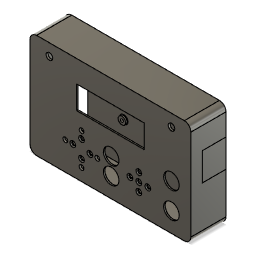
MegaElsCase (Autodesk Fusion 360 design; units mm, degrees)
Autodesk Fusion 360 part; units mm, degrees
sketch "Sketch1" plane through (0, 0, 0) normal (0, 0, 1) x (1, 0, 0)
  line L0 (0, 0) -> (160, 0)
  line L1 (160, 0) -> (160, 100)
  line L2 (160, 100) -> (0, 100)
  line L3 (0, 100) -> (0, 0)
  dimension "d1" = 160
  dimension "d2" = 100
  constraint horizontal L0
  constraint vertical L1
  constraint horizontal L2
  constraint vertical L3
  constraint coincident L0.start L3.end
  measures "d1" distance of L0.start L0.end
  measures "d2" distance of L0.start L2.end
extrude "Extrude1" add sketch "Sketch1" along normal blind 1.6 makes body 1
sketch "Sketch2" plane through (0, 0, 1.6) normal (0, 0, 1) x (1, 0, 0)
  line L0 (0, 100) -> (0, 0)
  line L1 (0, 0) -> (160, 0)
  line L2 (160, 0) -> (160, 100)
  line L3 (160, 100) -> (0, 100)
  line L4 (0, 0) -> (160, 0)
  line L5 (160, 0) -> (160, 100)
  line L6 (160, 100) -> (0, 100)
  line L7 (0, 100) -> (0, 0)
  line L8 (163, 103) -> (-3, 103)
  line L9 (-3, 103) -> (-3, -3)
  line L10 (-3, -3) -> (163, -3)
  line L11 (163, -3) -> (163, 103)
  line L12 (165, 105) -> (-5, 105)
  line L13 (-5, 105) -> (-5, -5)
  line L14 (-5, -5) -> (165, -5)
  line L15 (165, -5) -> (165, 105)
  circle A0 centre (15.5185, 92.5006) radius 3.5
  circle A1 centre (144.5011, 92.3883) radius 3.5
  circle A2 centre (80.8196, 33.8708) radius 8.25
  circle A3 centre (80.8007, 15.6853) radius 8.25
  circle A4 centre (144.4573, 43.0009) radius 8.25
  circle A5 centre (144.4275, 15.6835) radius 8.25
  line L16 (44.3, 81.7) -> (115.7, 81.7)
  line L17 (115.7, 81.7) -> (115.7, 57.3)
  line L18 (115.7, 57.3) -> (44.3, 57.3)
  line L19 (44.3, 57.3) -> (44.3, 81.7)
  circle A6 centre (49.4839, 33.8731) radius 2
  circle A7 centre (40.2387, 24.6612) radius 2
  circle A8 centre (58.3342, 24.6842) radius 2
  circle A9 centre (49.4706, 15.6511) radius 2
  circle A10 centre (49.4462, 7.8513) radius 2.5
  circle A11 centre (66.167, 24.6779) radius 2.5
  circle A12 centre (49.495, 41.543) radius 2.5
  circle A13 centre (32.3413, 24.6561) radius 2.5
  circle A14 centre (109.969, 33.8254) radius 2
  circle A15 centre (100.5787, 24.7006) radius 2
  circle A16 centre (109.9576, 24.7062) radius 2
  circle A17 centre (119.4752, 24.7124) radius 2
  circle A18 centre (109.9462, 15.6346) radius 2
  line L20 (32.3413, 24.6561) -> (119.4752, 24.7124) construction
  line L21 (49.495, 41.543) -> (49.4462, 7.8513) construction
  line L22 (109.969, 33.8254) -> (109.9462, 15.6346) construction
  circle A19 centre (2.54, 97.46) radius 2
  circle A20 centre (157.46, 97.46) radius 2
  circle A21 centre (157.46, 2.54) radius 2
  circle A22 centre (2.54, 2.54) radius 2
  circle A23 centre (2.54, 97.46) radius 4
  circle A24 centre (2.54, 2.54) radius 4
  circle A25 centre (157.46, 2.54) radius 4
  circle A26 centre (157.46, 97.46) radius 4
  line L23 (157.46, 6.54) -> (163, 6.54)
  line L24 (153.46, 2.54) -> (153.46, -3)
  line L25 (6.54, 2.54) -> (6.54, -3)
  line L26 (2.54, 6.54) -> (-3, 6.54)
  line L27 (2.54, 93.46) -> (-3, 93.46)
  line L28 (6.54, 97.46) -> (6.54, 103)
  line L29 (153.46, 97.46) -> (153.46, 103)
  line L30 (157.46, 93.46) -> (163, 93.46)
  circle A27 centre (100, 40) radius 2
  circle A28 centre (60, 40) radius 2
  circle A29 centre (60, 40) radius 4
  circle A30 centre (100, 40) radius 4
  line L31 (155.46, 100.9241) -> (155.46, 103)
  line L32 (160.9241, 95.46) -> (163, 95.46)
  line L33 (4.54, 100.9241) -> (4.54, 103)
  line L34 (-0.9241, 95.46) -> (-3, 95.46)
  line L35 (-0.9241, 4.54) -> (-3, 4.54)
  line L36 (4.54, -0.9241) -> (4.54, -3)
  line L37 (155.46, -0.9241) -> (155.46, -3)
  line L38 (160.9241, 4.54) -> (163, 4.54)
  dimension "d5" = 3
  dimension "d6" = 5
  dimension "d7" = 7
  dimension "d8" = 7
  dimension "d9" = 16.5
  dimension "d10" = 16.5
  dimension "d11" = 16.5
  dimension "d12" = 16.5
  dimension "d13" = 18.3
  dimension "d14" = 44.3
  dimension "d15" = 44.3
  dimension "d16" = 24.4
  dimension "d17" = 4
  dimension "d18" = 4
  dimension "d19" = 4
  dimension "d20" = 4
  dimension "d21" = 5
  dimension "d22" = 5
  dimension "d23" = 5
  dimension "d24" = 5
  dimension "d25" = 4
  dimension "d26" = 4
  dimension "d27" = 4
  dimension "d28" = 4
  dimension "d29" = 4
  dimension "d36" = 4
  dimension "d37" = 2.54
  dimension "d38" = 2.54
  dimension "d39" = 4
  dimension "d40" = 2.54
  dimension "d41" = 2.54
  dimension "d42" = 4
  dimension "d43" = 2.54
  dimension "d44" = 2.54
  dimension "d45" = 4
  dimension "d46" = 2.54
  dimension "d47" = 2.54
  dimension "d48" = 2
  dimension "d49" = 2
  dimension "d50" = 2
  dimension "d51" = 2
  dimension "d59" = 4
  dimension "d60" = 4
  dimension "d61" = 2
  dimension "d62" = 2
  dimension "d63" = 60
  dimension "d64" = 60
  dimension "d65" = 60
  dimension "d66" = 100
  dimension "d141" = 2
  dimension "d142" = 2
  dimension "d143" = 2
  dimension "d144" = 2
  dimension "d145" = 2
  dimension "d146" = 2
  dimension "d147" = 2
  dimension "d148" = 2
  constraint horizontal L4
  constraint vertical L5
  constraint horizontal L6
  constraint vertical L7
  constraint coincident L2.end L3.start
  constraint coincident L0.end L1.start
  constraint horizontal L16
  constraint vertical L17
  constraint horizontal L18
  constraint vertical L19
  constraint coincident A13.centre L20.start
  constraint coincident A17.centre L20.end
  constraint coincident A7.centre L20
  constraint coincident A11.centre L20
  constraint coincident A16.centre L20
  constraint coincident A12.centre L21.start
  constraint coincident A10.centre L21.end
  constraint coincident A6.centre L21
  constraint coincident A14.centre L22.start
  constraint coincident A18.centre L22.end
  constraint coincident A16.centre L22
  constraint coincident A25 L23.start
  constraint coincident L11 L23.end
  constraint tangent A25 L23
  constraint horizontal L23
  constraint coincident A25 L24.start
  constraint coincident L10 L24.end
  constraint perpendicular L10 L24
  constraint tangent A25 L24
  constraint coincident A24 L25.start
  constraint coincident L10 L25.end
  constraint coincident A24 L26.start
  constraint coincident L9 L26.end
  constraint perpendicular L9 L26
  constraint tangent A24 L26
  constraint tangent A24 L25
  constraint vertical L25
  constraint coincident A23 L27.start
  constraint coincident L9 L27.end
  constraint perpendicular L9 L27
  constraint coincident A23 L28.start
  constraint coincident L8 L28.end
  constraint perpendicular L8 L28
  constraint tangent A23 L28
  constraint tangent A23 L27
  constraint coincident A26 L29.start
  constraint coincident L8 L29.end
  constraint perpendicular L8 L29
  constraint coincident A26 L30.start
  constraint coincident L11 L30.end
  constraint perpendicular L11 L30
  constraint tangent A26 L30
  constraint tangent A26 L29
  constraint coincident A26 L31.start
  constraint coincident L8 L31.end
  constraint perpendicular L8 L31
  constraint coincident A26 L32.start
  constraint coincident L11 L32.end
  constraint perpendicular L11 L32
  constraint coincident A23 L33.start
  constraint coincident L8 L33.end
  constraint perpendicular L8 L33
  constraint coincident A23 L34.start
  constraint coincident L9 L34.end
  constraint perpendicular L9 L34
  constraint coincident A24 L35.start
  constraint coincident L9 L35.end
  constraint perpendicular L9 L35
  constraint coincident A24 L36.start
  constraint coincident L10 L36.end
  constraint perpendicular L10 L36
  constraint coincident A25 L37.start
  constraint coincident L10 L37.end
  constraint perpendicular L10 L37
  constraint coincident A25 L38.start
  constraint coincident L11 L38.end
  constraint perpendicular L11 L38
  measures "d7" diameter of A0
  measures "d8" diameter of A1
  measures "d9" diameter of A2
  measures "d10" diameter of A3
  measures "d11" diameter of A4
  measures "d12" diameter of A5
  measures "d13" distance of L6 L16
  measures "d14" distance of L7 L19
  measures "d15" distance of L5 L17
  measures "d16" distance of L16 L18
  measures "d17" diameter of A6
  measures "d18" diameter of A7
  measures "d19" diameter of A8
  measures "d20" diameter of A9
  measures "d21" diameter of A10
  measures "d22" diameter of A11
  measures "d23" diameter of A12
  measures "d24" diameter of A13
  measures "d25" diameter of A14
  measures "d26" diameter of A15
  measures "d27" diameter of A16
  measures "d28" diameter of A17
  measures "d29" diameter of A18
  measures "d36" diameter of A19
  measures "d37" distance of L6 A19.centre
  measures "d38" distance of L7 A19.centre
  measures "d39" diameter of A20
  measures "d40" distance of L6 A20.centre
  measures "d41" distance of L5 A20.centre
  measures "d42" diameter of A21
  measures "d43" distance of L5 A21.centre
  measures "d44" distance of L4 A21.centre
  measures "d45" diameter of A22
  measures "d46" distance of L4 A22.centre
  measures "d47" distance of L7 A22.centre
  measures "d48" distance of A19
  measures "d49" distance of A22
  measures "d50" distance of A21
  measures "d51" distance of A20
  measures "d59" diameter of A27
  measures "d60" diameter of A28
  measures "d61" distance of A28
  measures "d62" distance of A27
  measures "d63" distance of L5 A27.centre
  measures "d64" distance of L6 A27.centre
  measures "d65" distance of L6 A28.centre
  measures "d66" distance of L5 A28.centre
  measures "d141" distance of L30 L32
  measures "d142" distance of L29 L31
  measures "d143" distance of L27 L34
  measures "d144" distance of L28 L33
  measures "d145" distance of L26 L35
  measures "d146" distance of L25 L36
  measures "d147" distance of L23 L38
  measures "d148" distance of L24 L37
extrude "Extrude2" add sketch "Sketch2" along normal blind 2 from surface at 8.5 separate body contours L0 L3 L6 L7 A23 | L0 L3 L6 L7 A23 | L0 L7 A23 L27 | L0 L7 L9 A23 L27 L34 | L3 L6 L8 A23 L28 L33 | L3 L6 A23 L28 | L0 L1 L2 L3 L4 L5 L6 L7 A23 A24 A25 A26 L23 L24 L25 L26 L27 L28 L29 L30 | L0 L7 L9 L26 L27 | L8 L9 A23 L33 L34 | L3 L6 L8 L28 L29 | L0 L7 A24 L26 | L0 L7 L9 A24 L26 L35 | L3 L6 L8 A26 L29 L31 | L3 L6 A26 L29 | L0 L1 L4 L7 A24 | L0 L1 L4 L7 A24 | L2 L3 L5 L6 A26 | L2 L3 L5 L6 A26 | L9 L10 A24 L35 L36 | L1 L4 A24 L25 | L8 L11 A26 L31 L32 | L2 L5 A26 L30 | L1 L4 L10 A24 L25 L36 | L1 L4 L10 L24 L25 | L2 L5 L11 A26 L30 L32 | L2 L5 L11 L23 L30 | L1 L4 A25 L24 | L1 L4 L10 A25 L24 L37 | L2 L5 L11 A25 L23 L38 | L2 L5 A25 L23 | L1 L2 L4 L5 A25 | L1 L2 L4 L5 A25 | L10 L11 A25 L37 L38 | L12 L13 L14 L15 | A19 | A20 | A21 | A22 | A27 | A28 | A29 | A30 makes body 2
extrude "Extrude3" add sketch "Sketch2" against normal blind 35.1 from surface at 8.5 contours L12 L13 L14 L15 bodies 2
extrude "Extrude4" add sketch "Sketch2" along normal blind 8.5 contours L0 L3 L6 L7 A23 | L0 L3 L6 L7 A23 | L0 L7 A23 L27 | L0 L7 L9 A23 L27 L34 | L3 L6 L8 A23 L28 L33 | L3 L6 A23 L28 | L0 L7 A24 L26 | L0 L7 L9 A24 L26 L35 | L3 L6 L8 A26 L29 L31 | L3 L6 A26 L29 | L0 L1 L4 L7 A24 | L0 L1 L4 L7 A24 | L2 L3 L5 L6 A26 | L2 L3 L5 L6 A26 | L1 L4 A24 L25 | L2 L5 A26 L30 | L1 L4 L10 A24 L25 L36 | L2 L5 L11 A26 L30 L32 | L1 L4 A25 L24 | L1 L4 L10 A25 L24 L37 | L2 L5 L11 A25 L23 L38 | L2 L5 A25 L23 | L1 L2 L4 L5 A25 | L1 L2 L4 L5 A25 bodies 2
fillet "Fillet1" radius 5 4 edges at (163, 103, -7.45) (-3, 103, -7.45) (-3, -3, -7.45) (163, -3, -7.45) on bodies 2
fillet "Fillet2" radius 7 4 edges at (165, 105, -6.45) (-5, 105, -6.45) (165, -5, -6.45) (-5, -5, -6.45) on bodies 2
chamfer "Chamfer1" distance 1 angle 45 9 edges at (38.374, 25.3844, 12.1) (47.6192, 34.5963, 12.1) (56.4696, 25.4075, 12.1) (47.606, 16.3743, 12.1) (98.714, 25.4238, 12.1) (108.1043, 34.5486, 12.1) (108.0929, 25.4295, 12.1) (117.6105, 25.4356, 12.1) (108.0816, 16.3578, 12.1) on bodies 2
extrude "Extrude5" add sketch "Sketch2" along normal blind 8.5 contours A29 | A30 bodies 2
chamfer "Chamfer2" distance 2 angle 45 2 edges at (96.2707, 38.5535, 10.1) (56.2707, 38.5535, 10.1) on bodies 2
chamfer "Chamfer3" distance 0.5 angle 45 4 edges at (136.7358, 18.6668, 10.1) (136.7656, 45.9842, 10.1) (73.1279, 36.8541, 10.1) (73.109, 18.6686, 10.1) on bodies 2
chamfer "Chamfer4" distance 0.5 angle 45 8 edges at (163, 50, -25) (161.5355, 101.5355, -25) (80, 103, -25) (-1.5355, 101.5355, -25) (-3, 50, -25) (-1.5355, -1.5355, -25) (80, -3, -25) (161.5355, -1.5355, -25) on bodies 2
fillet "Fillet3" radius 1 4 edges at (163, 50, 10.1) (80, 103, 10.1) (-3, 50, 10.1) (80, -3, 10.1) on bodies 2
fillet "Fillet4" radius 0.5 4 edges at (80, 81.7, 10.1) (44.3, 69.5, 10.1) (80, 57.3, 10.1) (115.7, 69.5, 10.1) on bodies 2
sketch "Sketch3" plane through (0, 0, 1.6) normal (0, 0, 1) x (1, 0, 0)
  circle A0 centre (157.46, 97.46) radius 3
  circle A1 centre (2.54, 97.46) radius 3
  circle A2 centre (2.54, 2.54) radius 3
  circle A3 centre (157.46, 2.54) radius 3
  circle A4 centre (100, 40) radius 3
  circle A5 centre (60, 40) radius 3
  line L0 (158, 103) -> (2, 103)
  arc A6 (163, 98) -> (158, 103) centre (158, 98) ccw
  line L1 (163, 2) -> (163, 98)
  arc A7 (2, 103) -> (-3, 98) centre (2, 98) ccw
  line L2 (-3, 98) -> (-3, 2)
  arc A8 (-3, 2) -> (2, -3) centre (2, 2) ccw
  line L3 (2, -3) -> (158, -3)
  arc A9 (158, -3) -> (163, 2) centre (158, 2) ccw
  line L4 (144.9, 86) -> (144.9, 80.3818)
  arc A10 (144.9, 80.3818) -> (150.1, 80.3818) centre (147.5, 80.3818) ccw
  line L5 (150.1, 80.3818) -> (150.1, 86)
  arc A11 (150.1, 86) -> (144.9, 86) centre (147.5, 86) ccw
  line L6 (147.5, 86) -> (147.5, 80.3818) construction
  arc A12 (9.9, 80.3818) -> (15.1, 80.3818) centre (12.5, 80.3818) ccw
  line L7 (15.1, 80.3818) -> (15.1, 86)
  arc A13 (15.1, 86) -> (9.9, 86) centre (12.5, 86) ccw
  line L8 (9.9, 86) -> (9.9, 80.3818)
  line L9 (2, 105) -> (158, 105)
  circle A14 centre (147.5, 80.3818) radius 4.5
  circle A15 centre (12.5, 80.3818) radius 4.5
  circle A16 centre (157.46, 97.46) radius 1.55
  circle A17 centre (2.54, 97.46) radius 1.55
  circle A18 centre (2.54, 2.54) radius 1.55
  circle A19 centre (60, 40) radius 1.55
  circle A20 centre (100, 40) radius 1.55
  circle A21 centre (157.46, 2.54) radius 1.55
  circle A22 centre (2.54, 97.46) radius 4
  circle A23 centre (2.54, 2.54) radius 4
  circle A24 centre (60, 40) radius 4
  circle A25 centre (100, 40) radius 4
  circle A26 centre (157.46, 97.46) radius 4
  circle A27 centre (157.46, 2.54) radius 4
  line L10 (2, -2.65) -> (158, -2.65)
  arc A28 (158, -2.65) -> (162.65, 2) centre (158, 2) ccw
  line L11 (162.65, 2) -> (162.65, 98)
  arc A29 (162.65, 98) -> (158, 102.65) centre (158, 98) ccw
  line L12 (158, 102.65) -> (2, 102.65)
  arc A30 (2, 102.65) -> (-2.65, 98) centre (2, 98) ccw
  line L13 (-2.65, 98) -> (-2.65, 2)
  arc A31 (-2.65, 2) -> (2, -2.65) centre (2, 2) ccw
  line L14 (4.2879, 7.5347) -> (21.3888, 7.5347)
  line L15 (21.3888, 7.5347) -> (21.3888, 82.1018)
  line L16 (21.3888, 82.1018) -> (4.2879, 82.1018)
  line L17 (4.2879, 82.1018) -> (4.2879, 7.5347)
  point P0 (157.46, 97.46)
  point P1 (2.54, 97.46)
  point P2 (60, 40)
  point P3 (100, 40)
  point P4 (157.46, 2.54)
  point P5 (2.54, 2.54)
  dimension "d76" = 6
  dimension "d77" = 6
  dimension "d78" = 6
  dimension "d79" = 6
  dimension "d80" = 6
  dimension "d81" = 6
  dimension "d82" = 5.2
  dimension "d83" = 5.2
  dimension "d84" = 135
  dimension "d85" = 15.5
  dimension "d86" = 19
  dimension "d87" = 9
  dimension "d88" = 9
  dimension "d89" = 3.1
  dimension "d90" = 3.1
  dimension "d91" = 3.1
  dimension "d92" = 3.1
  dimension "d93" = 3.1
  dimension "d94" = 3.1
  dimension "d98" = 1
  dimension "d99" = 1
  dimension "d100" = 1
  dimension "d101" = 1
  dimension "d102" = 1
  dimension "d103" = 1
  dimension "d115" = -0.35
  constraint coincident P0 A0.centre
  constraint coincident P1 A1.centre
  constraint coincident P5 A2.centre
  constraint coincident P4 A3.centre
  constraint coincident P3 A4.centre
  constraint coincident P2 A5.centre
  constraint tangent L4 A10
  constraint tangent A10 L5
  constraint parallel L4 L5
  constraint tangent L5 A11
  constraint tangent L4 A11
  constraint vertical L6
  constraint tangent A12 L8
  constraint tangent A12 L7
  constraint parallel L7 L8
  constraint tangent L7 A13
  constraint tangent A13 L8
  constraint concentric A10 A14
  constraint concentric A12 A15
  constraint concentric A2 A18
  constraint concentric A4 A20
  constraint horizontal L14
  constraint vertical L15
  constraint horizontal L16
  constraint vertical L17
  measures "d76" diameter of A0
  measures "d77" diameter of A1
  measures "d78" diameter of A2
  measures "d79" diameter of A3
  measures "d80" diameter of A4
  measures "d81" diameter of A5
  measures "d82" diameter of A10
  measures "d83" diameter of A12
  measures "d84" distance of A10.centre A12.centre
  measures "d85" distance of L1 A10.centre
  measures "d86" distance of A11.centre L9
  measures "d87" diameter of A14
  measures "d88" diameter of A15
  measures "d89" diameter of A16
  measures "d90" diameter of A17
  measures "d91" diameter of A18
  measures "d92" diameter of A19
  measures "d93" diameter of A20
  measures "d94" diameter of A21
extrude "Extrude6" add sketch "Sketch3" against normal blind 3 from surface at -23.6 separate body contours L0 A6 L1 A7 L2 A8 L3 A9 | A15 L14 L15 L16 L17 | A22 | A23 | A24 | A25 | A26 | A27 | L10 A28 L11 A29 L12 A30 L13 A31 makes body 3
extrude "Extrude7" add sketch "Sketch3" along normal blind 2 from surface at -23.6 contours A0 | A1 | A2 | A3 | A4 | A5 | A22 | A23 | A24 | A25 | A26 | A27 bodies 3
fillet "Fillet8" radius 0.3 6 edges at (154.663, 98.5448, -22) (-0.257, 98.5448, -22) (-0.257, 3.6248, -22) (57.203, 41.0848, -22) (97.203, 41.0848, -22) (154.663, 3.6248, -22) on bodies 3
extrude "Extrude9" cut sketch "Sketch3" along normal up to surface (3 mm away) from surface at -26.6 contours A15 L14 L15 L16 L17 bodies 3
fillet "Fillet12" radius 1 4 edges at (4.2879, 7.5347, -23.5) (21.3888, 7.5347, -23.5) (21.3888, 82.1018, -23.5) (4.2879, 82.1018, -23.5) on bodies 3
fillet "Fillet13" radius 0.5 1 faces at (88.4794, 70.7168, -22) on bodies 3
sketch "Sketch4" plane through (163, 0, 0) normal (-1, 0, 0) x (0, 0, 1)
  line L0 (9.1, 6.54) -> (9.1, 93.46)
  line L1 (9.1, 93.46) -> (1.6, 93.46)
  line L2 (1.6, 93.46) -> (1.6, 95.46)
  line L3 (10.1, 98) -> (-24.5, 98)
  line L4 (-24.5, 98) -> (-24.5, 2)
  line L5 (-24.5, 2) -> (10.1, 2)
  line L6 (1.6, 6.54) -> (9.1, 6.54)
  line L7 (-25, 75) -> (0, 75)
  line L8 (0, 75) -> (0, 45)
  line L9 (0, 45) -> (-25, 45)
  line L10 (-25, 45) -> (-25, 75)
  line L11 (-24.5, 74.5) -> (-0.5, 74.5)
  line L12 (-0.5, 74.5) -> (-0.5, 45.5)
  line L13 (-0.5, 45.5) -> (-24.5, 45.5)
  line L14 (-24.5, 45.5) -> (-24.5, 74.5)
  line L15 (-24.5, 74.5) -> (-25, 74.5)
  line L16 (-24.5, 45.5) -> (-25, 45.5)
  line L17 (1.6, 95.46) -> (10.1, 95.46)
  line L18 (10.1, 95.46) -> (10.1, 98)
  line L19 (10.1, 2) -> (10.1, 4.54)
  line L20 (10.1, 4.54) -> (1.6, 4.54)
  line L21 (1.6, 4.54) -> (1.6, 6.54)
  point P0 (-25, 105)
  dimension "d135" = 25
  dimension "d136" = 30
  dimension "d137" = 30
  dimension "d138" = 0.5
  constraint horizontal L7
  constraint vertical L8
  constraint horizontal L9
  constraint vertical L10
  constraint coincident L10 L15.end
  constraint perpendicular L10 L15
  constraint coincident L10 L16.end
  constraint perpendicular L10 L16
  measures "d135" distance of L7.start L7.end
  measures "d136" distance of L7.start L9.end
  measures "d137" distance of P0 L7
extrude "Extrude11" cut sketch "Sketch4" against normal blind 1.5 contours L4 L9 L10 L16 | L4 L7 L8 L9 L11 L12 L13 | L4 L7 L10 L15 bodies 2
hidden bodies 1
equation "d34 = -8.5 mm - 1.6 mm - 20 mm - 2 mm - 3 mm"
equation "d85 = ( 166 / 2 ) * 1 mm - ( 135 / 2 ) * 1 mm"
equation "d95 = -1.6 mm - 20 mm - 2 mm"
named bodies: "PCB", "Main body", "Lid"
